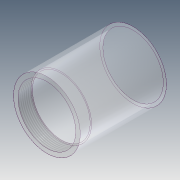
# Autodesk Inventor part: JF-AT-JC0005
Saved by Autodesk Inventor 2015 SP1 (Build 190203100, 203)
## iProperties
Created: 2010-03-12
Part Number: JF-AT-JC0005
Document SubType Name: Modeling
Designer: InventorUser
Density: 0.66 g/cm^3
Material: Acrylic, Clear
Description: Acrylic Tube Air Ball
Mass: 10.536 g
Surface Area: 141.448 cm^2
Volume: 15.9636 cm^3
Project: COMMON
Vendor: HHMI: JRC - ID&F
Appearance: Polycarbonate (Clear)
ALTERED ITEM PART NUMBER: N/A
ALTERED ITEM VENDOR: N/A
SPECIAL FINISH: NONE
SURFACE ROUGHNESS: N/A
LAB/DEPT: COMMON
REQUESTING SCIENTIST: COMMON
DESIGN DEPARTMENT: HHMI: JRC - ID&F
ALTERED ITEM DESCRIPTION: N/A
Revision Number: 0
Autodesk Inventor part; units mm, degrees
ref_plane "YZ Plane" through (0, 0, 0) normal (1, 0, 0) x (0, 1, 0)
ref_plane "XZ Plane" through (0, 0, 0) normal (0, 1, 0) x (-1, 0, 0)
ref_plane "XY Plane" through (0, 0, 0) normal (0, 0, 1) x (1, 0, 0)
sketch "Sketch1" plane through (0, 0, 0) normal (0, 0, 1) x (1, 0, 0)
  circle A0 centre (-13.5074, 0) radius 22.098
  point P0 (0, 0)
  dimension "d0" = 44.196
  constraints: 1 centre point
  measures "d0" diameter of A0
extrude "Extrusion1" add sketch "Sketch1" along normal blind 57.15
sketch "Sketch2" plane through (-13.5074, 0, 57.15) normal (0, 0, 1) x (1, 0, 0)
  circle A0 centre (0, 0) radius 22.098 projected
  point P0 (13.5074, 0)
  constraints: 1 coincident
hole "Hole1" at (-13.5074, 0, 57.15) direction (0, 0, -1) diameter 38.3032 depth 10.16 tip angle 118 thread size "1 9/16-20 UN" class "2B" standard "ANSI Unified Screw Threads"
sketch "Sketch3" plane through (-13.5074, 0, 0) normal (0, 0, -1) x (-1, 0, 0)
  circle A0 centre (0, 0) radius 22.098 projected
  circle A1 centre (0, 0) radius 20.0279
  point P0 (-13.5074, 0)
  dimension "d10" = 40.0558
  constraints: 1 centre point, 1 coincident
  measures "d10" diameter of A1
extrude "Extrusion2" cut sketch "Sketch3" against normal blind 47.625 contours A1
body "Solid1"
